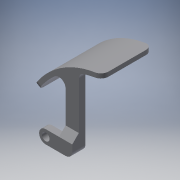
# Autodesk Inventor part: obstacle bumper
Saved by Autodesk Inventor 2016 (Build 200138000, 138)
## iProperties
Created: 2016-09-24
Part Number: obstacle bumper
Material: Generic
Document SubType Name: Modeling
Designer: benja
Density: 1 g/cm^3
Appearance: Default
Author: benja
Autodesk Inventor part; units mm, degrees
ref_plane "YZ Plane" through (0, 0, 0) normal (1, 0, 0) x (0, 1, 0)
ref_plane "XY Plane" through (0, 0, 0) normal (0, 0, 1) x (1, 0, 0)
sketch "Sketch1" plane through (0, 0, 0) normal (0, 0, 1) x (1, 0, 0)
  circle A0 centre (10.05, 11) radius 1.75
  arc A1 (13.575, 6.828427) -> (12.575, 7) centre (12.575, 4) ccw
  line L0 (13.575, 25.055513) -> (13.575, 6.828427)
  arc A2 (13.582607, 25.229787) -> (13.575, 25.055513) centre (15.575, 25.055513) ccw
  arc A3 (12.575, 25.055513) -> (13.582607, 25.229787) centre (12.575, 28.055513) ccw
  line L1 (7.525, 25.055513) -> (12.575, 25.055513)
  arc A4 (6.525, 25.227086) -> (7.525, 25.055513) centre (7.525, 28.055513) ccw
  line L2 (6.525, 6.828427) -> (6.525, 25.227086)
  arc A5 (7.525, 7) -> (6.525, 6.828427) centre (7.525, 4) ccw
  line L3 (12.575, 7) -> (7.525, 7)
  circle A6 centre (10.05, 21.055513) radius 1.75
  line L4 (10.05, 18.055513) -> (22.075, 18.055513)
  line L5 (22.075, 18.055513) -> (22.075, 56.065748)
  circle A7 centre (18.075, 30.055513) radius 1.75
  circle A8 centre (59, 30.055513) radius 1.75
  circle A9 centre (50.975, 2) radius 1.75
  circle A10 centre (10.05, 2) radius 1.75
  line L6 (3.525, -2) -> (3.525, 34.055513)
  arc A11 (3.525, -2) -> (63.525, -2) centre (33.525, 16.027756) ccw
  line L7 (63.525, 34.055513) -> (63.525, -2)
  arc A12 (63.525, 34.055513) -> (3.525, 34.055513) centre (33.525, 16.027756) ccw
  arc A13 (30.525, 56.680798) -> (-6.475, 36.055513) centre (29.281483, 15.411497) ccw
  arc A14 (30.525, 58.681663) -> (-8.207051, 37.055513) centre (29.281483, 15.411497) ccw
  line L8 (16.075, 54.530422) -> (16.075, 24.055513)
  line L9 (16.075, 24.055513) -> (10.05, 24.055513)
  arc A15 (10.05, 24.055513) -> (10.05, 18.055513) centre (10.05, 21.055513) ccw
  line L10 (-6.475, 36.055513) -> (-8.207051, 37.055513)
  line L11 (30.525, 56.680798) -> (30.525, 58.681663)
  line L12 (15.575, 28.055513) -> (15.575, 32.055513)
  point P0 (0, 0)
  point P1 (30.525, 57.681231)
  dimension "d0" = 6
  dimension "d1" = 6
  dimension "d2" = 3
  dimension "d3" = 2
  dimension "d4" = 2
  dimension "d5" = 0.5
  dimension "d6" = 60
  dimension "d22" = 10
  dimension "d23" = 2
  constraints: 12 end point, 8 point on circle, 3 centre point, 2 horizontal, 2 tangent, 1 coincident, 1 concentric, 1 line through centre, 1 midpoint, 1 perpendicular, 1 vertical, 1 vertical alignment
  measures "d0" distance between parallel lines of L4 L9
  measures "d1" distance between parallel lines of L5 L8
  measures "d2" distance from line of A11.centre L11
  measures "d4" radial gap between concentric circles of A13 A14
  measures "d5" distance between parallel lines of L8 L12
  measures "d6" angle of L11 L10
  measures "d22" distance from line of L6 L10.start
  measures "d23" vertical distance of L6.end L10.start
sketch "Sketch1 outline for Extrusion1" plane through (0, 0, 0) normal (0, 0, 1) x (1, 0, 0)
  arc A0 (-6.475, 36.055513) -> (16.075, 54.530422) centre (29.281483, 15.411497) cw
  line L0 (16.075, 54.530422) -> (16.075, 24.055513)
  line L1 (16.075, 24.055513) -> (10.05, 24.055513)
  arc A1 (10.05, 24.055513) -> (10.05, 18.055513) centre (10.05, 21.055513) ccw
  line L2 (10.05, 18.055513) -> (22.075, 18.055513)
  line L3 (22.075, 18.055513) -> (22.075, 56.065748)
  arc A2 (22.075, 56.065748) -> (30.525, 56.680798) centre (29.281483, 15.411497) cw
  line L4 (30.525, 56.680798) -> (30.525, 58.681663)
  arc A3 (30.525, 58.681663) -> (-8.207051, 37.055513) centre (29.281483, 15.411497) ccw
  line L5 (-8.207051, 37.055513) -> (-6.475, 36.055513)
  circle A4 centre (10.05, 21.055513) radius 1.75
extrude "Extrusion1" add sketch "Sketch1 outline for Extrusion1" along normal blind 6
sketch "Sketch2" plane through (0, 0, 0) normal (0, 0, -1) x (-1, 0, 0)
  circle A0 centre (-10.05, 21.055513) radius 1.75
  arc A1 (6.475, 36.055513) -> (-16.075, 54.530422) centre (-29.281483, 15.411497) ccw
  line L0 (8.207051, 37.055513) -> (6.475, 36.055513)
  arc A2 (8.207051, 37.055513) -> (-30.525, 58.681663) centre (-29.281483, 15.411497) ccw
  line L1 (-30.525, 56.680798) -> (-30.525, 58.681663)
  arc A3 (-22.075, 56.065748) -> (-30.525, 56.680798) centre (-29.281483, 15.411497) ccw
  line L2 (-22.075, 18.055513) -> (-22.075, 56.065748)
  line L3 (-10.05, 18.055513) -> (-22.075, 18.055513)
  arc A4 (-10.05, 18.055513) -> (-10.05, 24.055513) centre (-10.05, 21.055513) ccw
  line L4 (-16.075, 24.055513) -> (-10.05, 24.055513)
  line L5 (-16.075, 54.530422) -> (-16.075, 24.055513)
  line L6 (-16.075, 54.530422) -> (-16.075, 24.055513)
  line L7 (-10.05, 18.055513) -> (-22.075, 18.055513)
  line L8 (-19.575, 34.055513) -> (-12.575, 34.055513)
  line L9 (-22.075, 18.055513) -> (-22.075, 56.065748)
  line L10 (-16.075, 37.055513) -> (-22.075, 37.055513)
  line L11 (-22.075, 18.055513) -> (-22.075, 56.065748)
  line L12 (-16.075, 37.055513) -> (-16.075, 54.530422)
  line L13 (-22.075, 37.055513) -> (-22.075, 56.065748)
  point P0 (0, 0)
  point P1 (-16.0625, 18.055513)
  dimension "d20" = 3
  constraints: 6 end point, 2 collinear, 1 midpoint, 1 point on line
  measures "d20" distance between parallel lines of L8 L10
extrude "Extrusion2" add sketch "Sketch2" along normal blind 3 contours A1 L5 L10 L2 A3 L1 A2 L0
sketch "Sketch3" plane through (0, 0, 6) normal (0, 0, 1) x (1, 0, 0)
  line L0 (10.05, 18.055513) -> (22.075, 18.055513)
  line L1 (22.075, 18.055513) -> (22.075, 56.065748)
  arc A0 (30.525, 56.680798) -> (22.075, 56.065748) centre (29.281483, 15.411497) ccw
  line L2 (30.525, 56.680798) -> (30.525, 58.681663)
  arc A1 (30.525, 58.681663) -> (-8.207051, 37.055513) centre (29.281483, 15.411497) ccw
  line L3 (-8.207051, 37.055513) -> (-6.475, 36.055513)
  arc A2 (16.075, 54.530422) -> (-6.475, 36.055513) centre (29.281483, 15.411497) ccw
  line L4 (16.075, 54.530422) -> (16.075, 24.055513)
  line L5 (16.075, 24.055513) -> (10.05, 24.055513)
  arc A3 (10.05, 24.055513) -> (10.05, 18.055513) centre (10.05, 21.055513) ccw
  circle A4 centre (10.05, 21.055513) radius 1.75
  line L6 (5.525, 34.055513) -> (19.575, 34.055513)
  line L7 (16.075, 54.530422) -> (16.075, 24.055513)
  line L8 (22.075, 56.065748) -> (22.075, 18.055513)
  line L9 (16.075, 24.055513) -> (16.075, 54.530422)
  line L10 (16.075, 39.055513) -> (22.075, 39.055513)
  point P0 (0, 0)
  point P1 (22.075, 24.055513)
  point P2 (22.075, 34.055513)
  dimension "d19" = 5
  constraints: 4 point on line, 2 end point, 1 perpendicular
  measures "d19" distance between parallel lines of L6 L10
extrude "Extrusion3" cut sketch "Sketch3" against normal blind 3 contours L10 L4 A2 L3 A1 L2 A0 L1
sketch "Sketch4" plane through (0, 0, -3) normal (0, 0, -1) x (-1, 0, 0)
  arc A0 (6.475, 36.055513) -> (-16.075, 54.530422) centre (-29.281483, 15.411497) ccw
  line L0 (6.475, 36.055513) -> (8.207051, 37.055513)
  arc A1 (8.207051, 37.055513) -> (-30.525, 58.681663) centre (-29.281483, 15.411497) ccw
  line L1 (-30.525, 58.681663) -> (-30.525, 56.680798)
  arc A2 (-22.075, 56.065748) -> (-30.525, 56.680798) centre (-29.281483, 15.411497) ccw
  arc A3 (-16.075, 54.530422) -> (-22.075, 56.065748) centre (-29.281486, 15.411487) ccw
  arc A4 (-22.075, 56.065748) -> (-30.525, 56.680798) centre (-29.281483, 15.411497) ccw
  line L2 (-22.075, 56.065748) -> (-22.075, 37.055513)
  line L3 (-22.075, 37.055513) -> (-16.075, 37.055513)
  line L4 (-16.075, 37.055513) -> (-16.075, 54.530422)
  point P0 (0, 0)
  constraints: 2 point on circle, 1 centre point, 1 equal radius
extrude "Extrusion4" add sketch "Sketch4" along normal blind 20 contours A0 A3 A2 L1 A1 L0
fillet "Fillet1" radius 3 7 edges at (16.075, 54.5304, 0) (22.075, 56.0657, 0) (22.075, 18.0555, 3) (-7.341, 36.5555, 3) (-7.341, 36.5555, -23) (30.525, 57.6812, -23) (30.525, 57.6812, 3)
fillet "Fillet2" radius 3 4 edges at (19.075, 39.0555, 3) (19.075, 39.0555, 6) (19.075, 37.0555, -3) (19.075, 37.0555, 0)
ref_plane "Work Plane1" through (29.281483, 58.699528, 0) normal (0, 1, 0) x (-1, 0, 0)
sketch "Sketch6" plane through (0, 0, -3) normal (0, 0, -1) x (-1, 0, 0)
  line L0 (-16.075, 39.251665) -> (-22.075, 39.251665)
  line L1 (-16.075, 39.251665) -> (-16.075, 50.100446)
  arc A0 (-11.805166, 52.818446) -> (-16.075, 50.100446) centre (-13.075, 50.100446) ccw
  arc A1 (-16.075, 54.530422) -> (-22.075, 56.065748) centre (-29.281486, 15.411487) ccw
  arc A2 (-22.075, 53.467756) -> (-24.745407, 56.449595) centre (-25.075, 53.467756) ccw
  line L2 (-22.075, 53.467756) -> (-22.075, 39.251665)
  arc A3 (-3.525, 34.055513) -> (-63.525, 34.055513) centre (-33.525, 16.027756) ccw
  arc A4 (-16.075, 48.654394) -> (-22.075, 51.211524) centre (-33.525, 16.027756) ccw
  line L3 (-22.075, 53.467756) -> (-22.075, 42.055513)
  arc A5 (-16.075, 50.906081) -> (-22.075, 53.309085) centre (-33.525, 16.027756) ccw
  line L4 (-22.075, 51.211524) -> (-22.075, 53.309085)
  line L5 (-16.075, 50.906081) -> (-16.075, 48.654394)
  line L6 (-16.075, 39.251665) -> (-16.075, 50.100446)
  line L7 (-16.075, 42.055513) -> (-16.075, 50.100446)
  line L8 (-16.075, 50.100446) -> (-22.075, 53.309085)
  arc A6 (-11.805166, 52.818446) -> (-16.075, 54.530422) centre (-29.281483, 15.411497) ccw
  arc A7 (-22.075, 56.065748) -> (-24.745407, 56.449595) centre (-29.281483, 15.411497) ccw
  point P0 (0, 0)
  dimension "d37" = 2
  dimension "d38" = 2
  constraints: 6 end point, 4 point on circle, 3 collinear, 2 centre point, 2 coincident, 2 point on line
  measures "d37" radial gap between concentric circles of A3 A4
  measures "d38" radial gap between concentric circles of A4 A5
sketch "Sketch6 outline for Extrusion7" plane through (0, 0, -3) normal (0, 0, -1) x (-1, 0, 0)
  arc A0 (-16.075, 50.906081) -> (-22.075, 53.309085) centre (-33.525, 16.027756) ccw
  line L0 (-22.075, 53.309085) -> (-22.075, 39.251665)
  line L1 (-22.075, 39.251665) -> (-16.075, 39.251665)
  line L2 (-16.075, 39.251665) -> (-16.075, 50.906081)
extrude "Extrusion7" add sketch "Sketch6 outline for Extrusion7" along normal blind 8
fillet "Fillet6" radius 1 2 edges at (16.075, 45.0789, -11) (22.075, 46.2804, -11)
equation "\"d1\" = d0"
body "Solid1"
